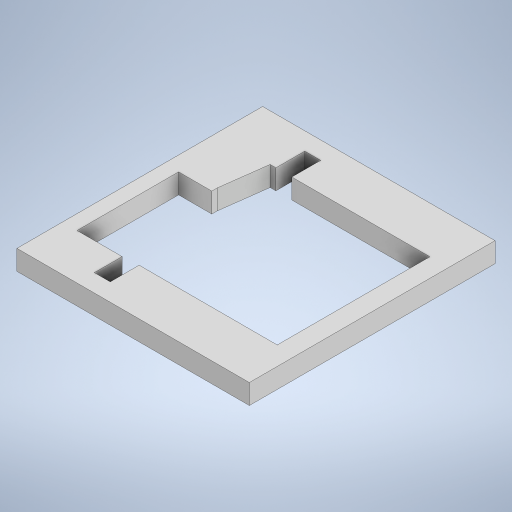
# Autodesk Inventor part: flipper_robot_v2_servo_side_profile
Saved by Autodesk Inventor 2023.1 (Build 271208000, 208)
## iProperties
Created: 2025-10-21
Part Number: flipper_robot_v2_servo_side_profile
Material: Generic
Document SubType Name: Modeling
Designer: Lars
Density: 1 g/cm^3
Appearance: Default
Author: Lars
Autodesk Inventor part; units mm, degrees
ref_plane "YZ Plane" through (0, 0, 0) normal (1, 0, 0) x (0, 1, 0)
ref_plane "XZ Plane" through (0, 0, 0) normal (0, 1, 0) x (-1, 0, 0)
ref_plane "XY Plane" through (0, 0, 0) normal (0, 0, 1) x (1, 0, 0)
sketch "Sketch1" plane through (0, 0, 0) normal (0, 1, 0) x (-1, 0, 0)
  line L0 (0, 0) -> (20.8, 0)
  line L1 (20.8, 0) -> (20.8, -22.6) construction
  line L2 (20.8, -22.6) -> (0, -22.6)
  line L3 (0, -22.6) -> (0, 0)
  line L4 (22.8, 4.35) -> (20.8, 4.35)
  line L5 (20.8, -26.95) -> (22.8, -26.95)
  line L6 (24.6, 0.15) -> (24.6, -22.45) construction
  line L7 (29.6, -14.7432) -> (24.6, -14.7432)
  line L8 (24.6, -14.7432) -> (24.6, 0.15) construction
  line L9 (24.6, -14.7432) -> (22.8, -14.7432) construction
  line L10 (24.6, -15.7432) -> (22.8, -15.7432) construction
  line L11 (24.6, -15.7432) -> (23.7, -22.6)
  line L12 (0, 0) -> (0, 7.2) construction
  line L13 (0, 7.2) -> (-3, 7.2) construction
  line L14 (-3, 7.2) -> (32, 7.2)
  line L15 (32, 7.2) -> (32, -29.8)
  line L16 (32, -29.8) -> (-3, -29.8)
  line L17 (-3, -29.8) -> (-3, 7.2)
  line L18 (24.6, 0.15) -> (24.6, -15.7432) construction
  line L19 (22.8, -22.6) -> (23.7, -22.6)
  line L20 (22.8, 0.1568) -> (22.8, 4.35)
  line L21 (22.8, -26.95) -> (22.8, -22.6)
  line L22 (24.6, -14.7432) -> (24.6, -15.7432)
  line L23 (20.8, 4.35) -> (20.8, 0)
  line L24 (20.8, -22.6) -> (20.8, -26.95)
  line L25 (29.6, 0.1568) -> (29.6, -14.7432)
  line L26 (22.8, 0.1568) -> (29.6, 0.1568)
  line L27 (29.8, 0.3568) -> (29.8, -14.9432)
  line L28 (29.8, -14.9432) -> (24.8, -14.9432)
  line L29 (24.8, -14.9432) -> (24.8, -15.7563)
  line L30 (24.8, -15.7563) -> (23.8755, -22.8)
  line L31 (23.8755, -22.8) -> (23, -22.8)
  line L32 (23, -22.8) -> (23, -27.15)
  line L33 (23, -27.15) -> (20.6, -27.15)
  line L34 (20.6, -27.15) -> (20.6, -22.8)
  line L35 (20.6, -22.8) -> (-0.2, -22.8)
  line L36 (-0.2, -22.8) -> (-0.2, 0.2)
  line L37 (-0.2, 0.2) -> (20.6, 0.2)
  line L38 (20.6, 0.2) -> (20.6, 4.55)
  line L39 (20.6, 4.55) -> (23, 4.55)
  line L40 (23, 4.55) -> (23, 0.3568)
  line L41 (23, 0.3568) -> (29.8, 0.3568)
  point P0 (20.8, -11.3)
  dimension "d0" = 20.8
  dimension "d1" = 22.6
  dimension "d2" = 2
  dimension "d5" = 22.6
  dimension "d8" = 1
  dimension "d9" = 7.2
  dimension "d10" = 3
  dimension "d11" = 35
  dimension "d12" = 37
  dimension "d16" = 2
  dimension "d19" = 4.35
  dimension "d26" = 6.8
  dimension "d27" = 0.9
  dimension "d28" = 14.9
  dimension "d29" = 5
  dimension "d32" = 0.2
  dimension "d35" = 4.35
  constraints: 84 end point, 17 parallel, 13 perpendicular, 4 horizontal, 2 collinear, 2 vertical, 1 midpoint, 1 point on line, 14 other
  measures "d0" distance of L1.end L2.end
  measures "d1" distance of L0.end L1.end
  measures "d2" distance of L5.start L5.end
  measures "d5" distance of L6.start L6.end
  measures "d8" distance between parallel lines of L9 L10
  measures "d9" distance of L0.start L12.end
  measures "d10" distance of L12.end L13.end
  measures "d11" distance of L15.end L16.end
  measures "d12" distance of L14.end L15.end
  measures "d16" distance of L4.start L4.end
  measures "d19" distance of L4.end L0.end
  measures "d26" distance of L20.start L25.start
  measures "d27" distance of L19.start L11.end
  measures "d28" distance between parallel lines of L7 L26
  measures "d29" distance of L7.start L7.end
  measures "d32" distance between parallel lines of L26 L41
  measures "d35" distance of L1.end L5.start
extrude "Extrusion5" add sketch "Sketch1" along normal blind 3 contours L14 L15 L16 L17
body "Solid5"
